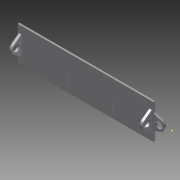
# Autodesk Inventor part: ForceMeterCasing
Saved by Autodesk Inventor 2012 SP2 (Build 160219200, 219)
## iProperties
Created: 2014-02-08
Part Number: ForceMeterCasing
Material: Default
Document SubType Name: Modeling
Designer: 1
Density: 1 g/cm^3
Author: 1
Autodesk Inventor part; units mm, degrees
ref_plane "YZ Plane" through (0, 0, 0) normal (1, 0, 0) x (0, 1, 0)
ref_plane "XZ Plane" through (0, 0, 0) normal (0, 1, 0) x (-1, 0, 0)
ref_plane "XY Plane" through (0, 0, 0) normal (0, 0, 1) x (1, 0, 0)
sketch "Sketch1" plane through (0, 0, 0) normal (0, 0, 1) x (1, 0, 0)
  point P0 (0, 0)
sketch "Sketch2" plane through (0, 0, 0) normal (0, 0, 1) x (1, 0, 0)
  line L0 (-30, 35) -> (-310, 35)
  line L1 (-310, 35) -> (-310, -35)
  line L2 (-310, -35) -> (-30, -35)
  line L3 (-30, -35) -> (-30, 35)
  line L4 (-310, 35) -> (-30, -35) construction
  line L5 (-30, 35) -> (-310, -35) construction
  line L6 (0, 0) -> (-620.4685, 0)
  point P0 (-170, 0)
  dimension "d0" = 280
  dimension "d1" = 70
  dimension "d2" = 30
  constraints: 14 end point, 2 parallel, 2 perpendicular, 1 horizontal, 1 midpoint, 1 point on line
  measures "d0" distance of L1.end L2.end
  measures "d1" distance of L0.end L1.end
  measures "d2" distance from line of L6.start L3
extrude "Extrusion1" add sketch "Sketch2" along normal blind 3.65
sketch "Sketch3" plane through (0, 0, 3.65) normal (0, 0, 1) x (1, 0, 0)
  line L0 (-30, 35) -> (-30, -35) projected
  line L1 (-310, -35) -> (-310, 35) projected
  line L2 (-30, 0) -> (-310, 0) construction
  line L3 (-42.4613, 25) -> (-37.4613, 25)
  line L4 (-37.4613, 25) -> (-37.4613, -25)
  line L5 (-37.4613, -25) -> (-42.4613, -25)
  line L6 (-42.4613, -25) -> (-42.4613, 25)
  line L7 (-37.4613, 25) -> (-42.4613, -25) construction
  line L8 (-42.4613, 25) -> (-37.4613, -25) construction
  point P0 (0, 0)
  point P1 (-39.9613, 0)
  dimension "d5" = 5
  dimension "d6" = 50
  constraints: 14 end point, 3 midpoint, 2 parallel, 1 horizontal, 1 perpendicular, 1 point on line
  measures "d5" distance of L4.end L5.end
  measures "d6" distance of L5.end L3.start
extrude "Extrusion2" add sketch "Sketch3" along normal blind 35.4
sketch "Sketch4" plane through (-42.4613, -25, 3.65) normal (-1, 0, 0) x (0, 0, 1)
  line L0 (35.4, 0) -> (35.4, 50) projected
  line L1 (0, 50) -> (35.4, 50) projected
  line L2 (0, 0) -> (0, 50) projected
  line L3 (0, 0) -> (35.4, 0) projected
  circle A0 centre (10, 25) radius 10 construction
  line L4 (35.4, 25) -> (-31.6063, 25)
  line L5 (0, 44.8702) -> (15.9582, 33.0312)
  line L6 (0, 5.1298) -> (15.9582, 16.9688)
  circle A1 centre (10, 25) radius 6.4008
  arc A2 (15.9582, 16.9688) -> (15.9582, 33.0312) centre (10, 25) ccw
  line L7 (0, 60) -> (0, -10) projected
  line L8 (0, 50) -> (35.4, 0) construction
  line L9 (35.4, 50) -> (0, 0) construction
  line L10 (0, -10) -> (0, 60) projected
  point P0 (-3.65, 25)
  point P1 (17.7, 25)
  point P2 (17.7, 25)
  dimension "d9" = 20
  constraints: 10 end point, 5 point on line, 3 midpoint, 2 centre point, 2 coincident, 2 point on circle, 2 symmetric about line, 1 perpendicular, 1 vertical, 4 other
extrude "Extrusion3" cut sketch "Sketch4" against normal through all contours L3 L2 L6 A2 L4 L0 | L4 A2 L5 L2 L1 L0 | A1 L4 | L4 A1
pattern_linear "Rectangular Pattern1" count 2 spacing 265 along (-1, 0, 0) of "Extrusion3", "Extrusion2"
sketch "Sketch5" plane through (0, 0, 3.65) normal (0, 0, 1) x (1, 0, 0)
  line L0 (-30, -35) -> (-310, -35) projected
  line L1 (-115.953, 3.5653) -> (-116.904, 3.5653)
  line L2 (-116.904, 3.5653) -> (-116.904, -30.6059)
  line L3 (-116.904, -30.6059) -> (-115.953, -30.6059)
  line L4 (-115.953, -30.6059) -> (-115.953, 3.5653)
  line L5 (-85.953, 3.5653) -> (-86.904, 3.5653)
  line L6 (-86.904, 3.5653) -> (-86.904, -30.6059)
  line L7 (-86.904, -30.6059) -> (-85.953, -30.6059)
  line L8 (-85.953, -30.6059) -> (-85.953, 3.5653)
  line L9 (-55.953, 3.5653) -> (-56.904, 3.5653)
  line L10 (-56.904, 3.5653) -> (-56.904, -30.6059)
  line L11 (-56.904, -30.6059) -> (-55.953, -30.6059)
  line L12 (-55.953, -30.6059) -> (-55.953, 3.5653)
  line L13 (-25.953, 3.5653) -> (-26.904, 3.5653)
  line L14 (-26.904, 3.5653) -> (-26.904, -30.6059)
  line L15 (-26.904, -30.6059) -> (-25.953, -30.6059)
  line L16 (-25.953, -30.6059) -> (-25.953, 3.5653)
  line L17 (4.047, 3.5653) -> (3.096, 3.5653)
  line L18 (3.096, 3.5653) -> (3.096, -30.6059)
  line L19 (3.096, -30.6059) -> (4.047, -30.6059)
  line L20 (4.047, -30.6059) -> (4.047, 3.5653)
  line L21 (34.047, 3.5653) -> (33.096, 3.5653)
  line L22 (33.096, 3.5653) -> (33.096, -30.6059)
  line L23 (33.096, -30.6059) -> (34.047, -30.6059)
  line L24 (34.047, -30.6059) -> (34.047, 3.5653)
  point P0 (0, 0)
  dimension "d17" = 30
  constraints: 48 end point, 2 horizontal, 2 parallel, 1 perpendicular, 40 other
  measures "d17" distance of L3.end L8.start
extrude "Extrusion4" cut sketch "Sketch5" against normal blind 0.25 contours L4 L3 L2 L1
pattern_linear "Rectangular Pattern2" count 6 spacing 30 along (-1, 0, 0) of "Extrusion4"
sketch "Sketch6" plane through (-30, -35, 0) normal (1, 0, 0) x (0, 0, -1)
  line L0 (-3.65, 70) -> (-3.65, 0) projected
  line L1 (0, 0) -> (-3.65, 0) projected
  line L2 (0, 0) -> (0, 70) projected
  line L3 (0, 70) -> (-3.65, 70) projected
  point P0 (0, 35)
extrude "Extrusion5" add sketch "Sketch6" along normal blind 17.7125
sketch "Sketch7" plane through (0, 0, 3.65) normal (0, 0, 1) x (1, 0, 0)
  line L0 (-266.904, -30.6059) -> (-266.904, 3.5653) projected
  line L1 (-266.904, 3.5653) -> (-265.953, 3.5653) projected
  line L2 (-265.953, 3.5653) -> (-265.953, -30.6059) projected
  line L3 (-265.953, -30.6059) -> (-266.904, -30.6059) projected
  line L4 (-236.904, -30.6059) -> (-236.904, 3.5653) projected
  line L5 (-236.904, 3.5653) -> (-235.953, 3.5653) projected
  line L6 (-235.953, 3.5653) -> (-235.953, -30.6059) projected
  line L7 (-235.953, -30.6059) -> (-236.904, -30.6059) projected
  line L8 (-206.904, -30.6059) -> (-206.904, 3.5653) projected
  line L9 (-206.904, 3.5653) -> (-205.953, 3.5653) projected
  line L10 (-205.953, 3.5653) -> (-205.953, -30.6059) projected
  line L11 (-205.953, -30.6059) -> (-206.904, -30.6059) projected
  line L12 (-176.904, -30.6059) -> (-176.904, 3.5653) projected
  line L13 (-176.904, 3.5653) -> (-175.953, 3.5653) projected
  line L14 (-175.953, 3.5653) -> (-175.953, -30.6059) projected
  line L15 (-175.953, -30.6059) -> (-176.904, -30.6059) projected
  line L16 (-146.904, -30.6059) -> (-146.904, 3.5653) projected
  line L17 (-146.904, 3.5653) -> (-145.953, 3.5653) projected
  line L18 (-145.953, 3.5653) -> (-145.953, -30.6059) projected
  line L19 (-145.953, -30.6059) -> (-146.904, -30.6059) projected
  line L20 (-116.904, -30.6059) -> (-116.904, 3.5653) projected
  line L21 (-116.904, 3.5653) -> (-115.953, 3.5653) projected
  line L22 (-115.953, 3.5653) -> (-115.953, -30.6059) projected
  line L23 (-115.953, -30.6059) -> (-116.904, -30.6059) projected
  line L24 (-302.4613, 19.8702) -> (-302.4613, -19.8702) projected
  line L25 (-307.4613, -19.8702) -> (-302.4613, -19.8702) projected
  line L26 (-307.4613, -19.8702) -> (-307.4613, 19.8702) projected
  line L27 (-307.4613, 19.8702) -> (-302.4613, 19.8702) projected
  line L28 (-310, 35) -> (-12.2875, 35) projected
  line L29 (-310, -35) -> (-310, 35) projected
  line L30 (-12.2875, -35) -> (-310, -35) projected
  line L31 (-12.2875, -35) -> (-12.2875, 35) projected
  line L32 (-42.4613, -19.8702) -> (-42.4613, 19.8702) projected
  line L33 (-42.4613, 19.8702) -> (-37.4613, 19.8702) projected
  line L34 (-37.4613, 19.8702) -> (-37.4613, -19.8702) projected
  line L35 (-42.4613, -19.8702) -> (-37.4613, -19.8702) projected
  line L36 (-12.2875, 35) -> (-12.2875, -35)
  circle A0 centre (-23.1854, 0) radius 10.8979 construction
  line L37 (-12.2875, -35) -> (-12.2875, 35) projected
  line L38 (-34.0833, 15.009) -> (-19.8116, 10.3625)
  line L39 (-34.0833, 15.009) -> (-34.0833, 35)
  line L40 (-12.2875, 35) -> (-12.2875, 0)
  arc A1 (-12.2875, 0) -> (-19.8116, 10.3625) centre (-23.1854, 0) ccw
  line L41 (-310, 0) -> (-198.3644, 0)
  circle A2 centre (-23.1854, 0) radius 10.8979 construction
  line L42 (-34.0833, -15.009) -> (-19.8116, -10.3625)
  line L43 (-34.0833, -15.009) -> (-34.0833, -35)
  arc A3 (-19.8116, -10.3625) -> (-12.2875, 0) centre (-23.1854, 0) ccw
  line L44 (-34.0833, 15.009) -> (-34.0833, 35)
  line L45 (-12.2875, 35) -> (-12.2875, 0)
  line L46 (-12.2875, -35) -> (-34.0833, -35)
  circle A4 centre (-23.1854, 0) radius 6.826
  constraints: 20 end point, 8 point on circle, 6 tangent, 5 centre point, 3 coincident, 3 collinear, 3 symmetric about line, 2 midpoint, 1 perpendicular, 1 point on line, 2 other
extrude "Extrusion6" cut sketch "Sketch7" against normal through all contours L28 L31 A1 L38 L39 | L31 L30 L43 L42 A3 | A4
fillet "Fillet1" radius 2 4 edges at (-39.9613, -19.8702, 3.65) (-39.9613, 19.8702, 3.65) (-304.9613, -19.8702, 3.65) (-304.9613, 19.8702, 3.65)
body "Solid1"
